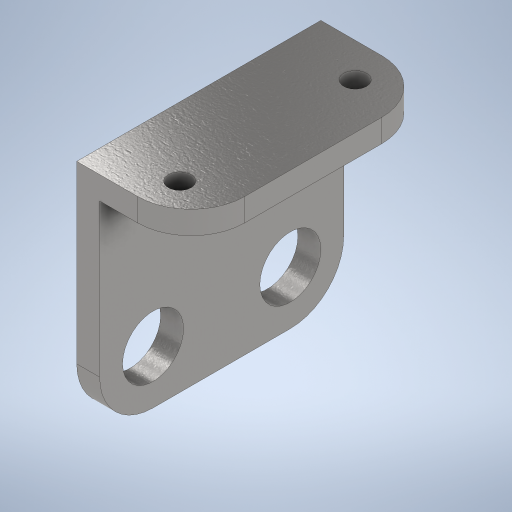
# Autodesk Inventor part: HUDSON-1-76
Saved by Autodesk Inventor 2024.2 (Build 282272000, 272)
## iProperties
Created: 2024-09-29
Part Number: HUDSON-1-76
Material: Generic
Document SubType Name: Modeling
Designer: melim
Density: 1 g/cm^3
Appearance: Galvanized
Author: melim
Autodesk Inventor part; units mm, degrees
ref_plane "YZ Plane" through (0, 0, 0) normal (1, 0, 0) x (0, 1, 0)
ref_plane "XZ Plane" through (0, 0, 0) normal (0, 1, 0) x (-1, 0, 0)
ref_plane "XY Plane" through (0, 0, 0) normal (0, 0, 1) x (1, 0, 0)
sketch "Sketch1" plane through (0, 0, 0) normal (0, 0, 1) x (1, 0, 0)
  line L0 (0, 0) -> (0, 30)
  line L1 (0, 30) -> (15, 30)
  line L2 (15, 30) -> (15, 27)
  line L3 (15, 27) -> (3, 27)
  line L4 (3, 27) -> (3, 0)
  line L5 (3, 0) -> (0, 0)
  dimension "d0" = 30
  dimension "d1" = 12
  dimension "d2" = 3
  dimension "d3" = 3
  constraints: 12 end point, 4 perpendicular, 1 parallel, 1 vertical
  measures "d0" distance of L0.start L0.end
  measures "d1" distance of L2.end L3.end
  measures "d2" distance between parallel lines of L1 L3
  measures "d3" distance between parallel lines of L0 L4
extrude "Extrusion1" add sketch "Sketch1" along normal blind 32
fillet "Fillet1" radius 7 2 edges at (1.5, 0, 32) (1.5, 0, 0)
sketch "Sketch2" plane through (3, 27, 32) normal (1, 0, 0) x (0, 0, -1)
  line L0 (0, -20) -> (0, 0) projected
  line L1 (32, 3) -> (0, 3) projected
  point P0 (32, -27)
  point P1 (7, -20)
  point P2 (25, -20)
  dimension "d7" = 18
  dimension "d8" = 7
  dimension "d9" = 23
  dimension "d10" = 23
  measures "d7" distance of point (7, -20) point (25, -20)
  measures "d8" distance from line of L0 point (7, -20)
  measures "d9" distance from line of L1 point (7, -20)
  measures "d10" distance from line of L1 point (25, -20)
hole "Hole1" at (3, 7, 25) at (3, 7, 7) direction (-1, 0, 0) diameter 8 end through all
sketch "Sketch3" plane through (0, 30, 0) normal (0, 1, 0) x (1, 0, 0)
  line L0 (15, 0) -> (0, 0) projected
  line L1 (0, 0) -> (0, -32) projected
  point P0 (9, -27.5)
  point P1 (9, -4.5)
  dimension "d18" = 23
  dimension "d19" = 4.5
  dimension "d20" = 9
  dimension "d21" = 9
  measures "d18" distance of point (9, -27.5) point (9, -4.5)
  measures "d19" distance from line of L0 point (9, -4.5)
  measures "d20" distance from line of L1 point (9, -27.5)
  measures "d21" distance from line of L1 point (9, -4.5)
hole "Hole2" at (9, 30, 27.5) at (9, 30, 4.5) direction (0, -1, 0) diameter 3 end through all
fillet "Fillet2" radius 7 2 edges at (15, 28.5, 0) (15, 28.5, 32)
body "Solid1"
